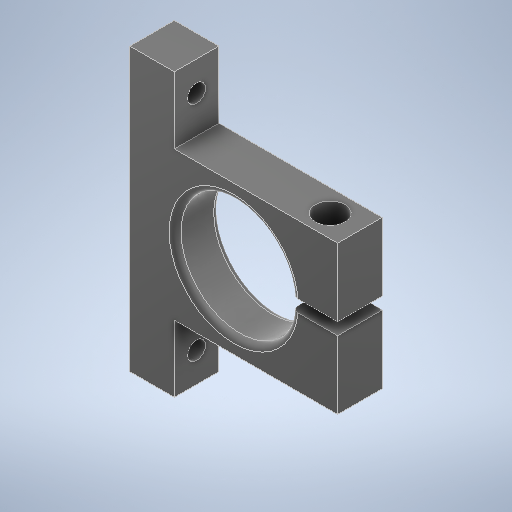
# Autodesk Inventor part: Magazine_Holder
Saved by Autodesk Inventor 2025.1 (Build 291241020, 241B)
## iProperties
Created: 2024-11-13
Part Number: Magazine_Holder
Material: PC/ABS Plastic
Document SubType Name: Modeling
Designer: leon-
Density: 1.1 g/cm^3
Appearance: Smooth - Black
Author: leon-
## iProperties of the stored document Magazine_Holder_3DPrint.ipt
Created: 2024-11-17
Part Number: Magazine_Holder_3DPrint
Material: Generic
Document SubType Name: Modeling
Designer: leon-
Density: 1 g/cm^3
Appearance: Default
Author: leon-
Autodesk Inventor part; units mm, degrees
ref_plane "YZ Plane" through (0, 0, 0) normal (1, 0, 0) x (0, 1, 0)
ref_plane "XZ Plane" through (0, 0, 0) normal (0, 1, 0) x (-1, 0, 0)
ref_plane "XY Plane" through (0, 0, 0) normal (0, 0, 1) x (1, 0, 0)
sketch "Sketch1" plane through (0, 0, 0) normal (0, 0, 1) x (1, 0, 0)
  line L0 (0, 0) -> (70, 0)
  line L1 (70, 0) -> (70, 25)
  line L2 (70, 25) -> (15, 25)
  line L3 (15, 25) -> (15, 47.5)
  line L4 (15, 47.5) -> (0, 47.5)
  line L5 (0, 47.5) -> (0, 0)
  point P0 (15, 36.25)
  point P1 (7.5, 47.5)
  dimension "d0" = 15
  dimension "d1" = 25
  dimension "d2" = 47.5
  dimension "d24" = 55
  constraints: 12 end point, 5 perpendicular, 2 midpoint, 1 horizontal
  measures "d0" distance from line of point (15, 36.25) L5
  measures "d1" distance between parallel lines of L0 L2
  measures "d2" distance from line of L0 point (7.5, 47.5)
  measures "d24" distance between parallel lines of L1 L3
extrude "Extrusion1" add sketch "Sketch1" along normal blind 15
mirror "Mirror1" about plane through (0, 0, 0) normal (0, 1, 0) of "Extrusion1"
sketch "Sketch2" plane through (0, 0, 15) normal (0, 0, 1) x (1, 0, 0)
  circle A0 centre (35, 0) radius 19.75
  line L0 (-14, 0) -> (84, 0) projected
  line L1 (70, 25) -> (70, -25) projected
  line L2 (70, 2) -> (35, 2)
  line L3 (35, 2) -> (35, -2)
  line L4 (35, -2) -> (70, -2)
  line L5 (70, -2) -> (70, 2)
  point P0 (0, 0)
  point P1 (52.5, 2)
  point P2 (54.6485, 2)
  point P3 (54.6485, -2)
  dimension "d6" = 39.5
  dimension "d7" = 35
  dimension "d8" = 4
  dimension "d9" = 2
  constraints: 8 end point, 3 midpoint, 2 parallel, 1 centre point, 1 horizontal, 1 perpendicular, 1 point on line
  measures "d6" diameter of A0
  measures "d7" distance from line of L1 A0.centre
  measures "d8" distance between parallel lines of L4 L2
  measures "d9" distance from line of L0 point (52.5, 2)
extrude "Extrusion2" cut sketch "Sketch2" against normal through all
sketch "Sketch3" plane through (15, 25, 0) normal (0, 1, 0) x (1, 0, 0)
  line L0 (55, 0) -> (0, 0) projected
  line L1 (55, 0) -> (55, -15) projected
  point P0 (-15, 0)
  point P1 (45, -7.5)
  dimension "d12" = 7.5
  dimension "d13" = 10
  measures "d12" distance from line of L0 point (45, -7.5)
  measures "d13" distance from line of L1 point (45, -7.5)
hole "Hole1" at (60, 25, 7.5) direction (0, -1, 0) diameter 6 end through all
sketch "Sketch4" plane through (15, 25, 0) normal (0, 1, 0) x (1, 0, 0)
  circle A0 centre (45, -7.5) radius 3 projected
  circle A1 centre (45, -7.5) radius 5
  point P0 (-15, 0)
  dimension "d21" = 10
  constraints: 1 centre point, 1 coincident
  measures "d21" diameter of A1
extrude "Extrusion3" cut sketch "Sketch4" against normal blind 15
mirror "Mirror2" about plane through (0, 0, 0) normal (0, 1, 0) of "Extrusion3"
sketch "Sketch5" plane through (15, 25, 0) normal (1, 0, 0) x (0, 0, -1)
  line L0 (0, 0) -> (0, 22.5) projected
  line L1 (0, 22.5) -> (-15, 22.5) projected
  point P0 (0, -25)
  point P1 (-7.5, 12.5)
  point P2 (0, 11.25)
  dimension "d26" = 7.5
  dimension "d34" = 10
  constraints: 1 midpoint
  measures "d26" distance from line of L0 point (-7.5, 12.5)
  measures "d34" distance from line of L1 point (-7.5, 12.5)
hole "Hole2" at (15, 37.5, 7.5) direction (-1, 0, 0) diameter 6 end through all
mirror "Mirror3" about plane through (0, 0, 0) normal (0, 1, 0) of "Hole2"
fillet "Fillet1" radius 2 2 edges at (15.25, 0, 15) (15.25, 0, 0)
equation "\"d9\" = 0.5 * d8"
body "Solid1"
